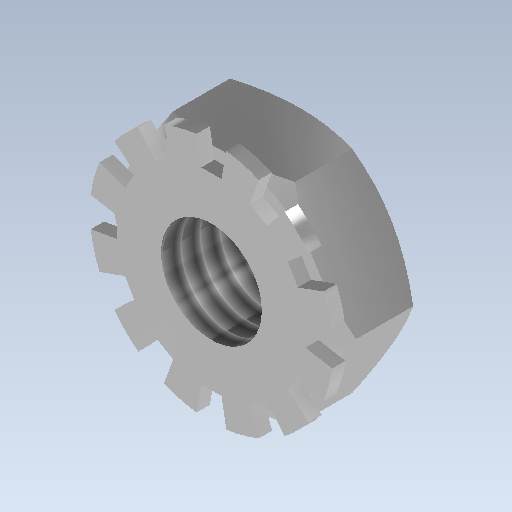
# Autodesk Inventor part: 275-1026
Saved by Autodesk Inventor 2020.2 (Build 242310000, 310)
## iProperties
Created: 2012-04-11
Part Number: 275-1026
Material: Stainless Steel, 440C
Document SubType Name: Modeling
Designer: Autodesk Inc.
Density: 7.75 g/cm^3
Catalog Web Link: http://www.vexrobotics.com/nuts-8-32.html
Vendor: VEX
Appearance: Black Chrome
Company: Autodesk Inc.
Category: Structure
Control State: 0
Master: False
Checked Out: False
Shininess: 70.0
Length Units: 11272
Angle Units: 11279
Time Units: 11290
Mass Units: 11286
Length Display Precision: 4
Angle Display Precision: 2
Compacted: True
Density: 7.75
Volumn: 0.07820028819372563
Area: 1.577785810948415
PropertySet Name: Model Information
Author: Autodesk Inc.
Autodesk Inventor part; units mm, degrees
ref_plane "YZ Plane" through (0, 0, 0) normal (1, 0, 0) x (0, 1, 0)
ref_plane "XZ Plane" through (0, 0, 0) normal (0, 1, 0) x (-1, 0, 0)
ref_plane "XY Plane" through (0, 0, 0) normal (0, 0, 1) x (1, 0, 0)
sketch "Sketch2" plane through (0, 0, 0) normal (0, 0, 1) x (1, 0, 0)
  circle A0 centre (0, 0) radius 5.0417 construction
  line L0 (-2.5209, 4.3663) -> (2.5209, 4.3663)
  line L1 (2.5209, 4.3663) -> (5.0417, 0)
  line L2 (5.0417, 0) -> (2.5209, -4.3663)
  line L3 (2.5209, -4.3663) -> (-2.5209, -4.3663)
  line L4 (-2.5209, -4.3663) -> (-5.0417, 0)
  line L5 (-5.0417, 0) -> (-2.5209, 4.3663)
  line L6 (0, 7.0584) -> (0, -7.0584) projected
  line L7 (-7.0584, 0) -> (7.0584, 0) projected
  dimension "Flats" = 8.7325
  constraints: 12 end point, 6 point on circle, 3 equal length, 2 midpoint, 1 centre point, 1 coincident, 1 parallel, 1 other
  measures "Flats" distance between parallel lines of L1 L4
extrude "Extrusion2" add sketch "Sketch2" along normal blind 3.1369
sketch "Sketch4" plane through (0, 0, 0) normal (1, 0, 0) x (0, 1, 0)
  line L0 (0, 3.1369) -> (4.3663, 3.1369) projected
  line L1 (4.3663, 3.1369) -> (8.7325, 0.616)
  line L2 (0, 0) -> (0, 3.1369) projected
  line L3 (4.3663, 3.1369) -> (8.7325, 3.1369)
  line L4 (8.7325, 0.616) -> (8.7325, 3.1369)
  dimension "d6" = 8.7325
  dimension "d7" = 30
  constraints: 6 end point, 2 perpendicular
  measures "d6" distance from line of L2 L1.end
  measures "d7" angle of L3 L1
revolve "Revolution1" cut sketch "Sketch4" angle 360 about axis through (0, 0, 0) along (0, 0, 1)
ref_plane "Work Plane1" through (0, 0, 1.5685) normal (0, 0, 1) x (1, 0, 0)
mirror "Mirror1" about plane through (0, 0, 1.5685) normal (0, 0, 1) of "Revolution1"
sketch "Sketch5" plane through (0, 0, 3.1369) normal (0, 0, 1) x (1, 0, 0)
  arc A0 (0, 4.3663) -> (-3.7813, 2.1831) centre (0, 0) ccw projected
  circle A1 centre (0, 0) radius 2.0828
  dimension "HoleDiam" = 4.1656
  constraints: 1 centre point, 1 coincident
  measures "HoleDiam" diameter of A1
extrude "Extrusion3" cut sketch "Sketch5" against normal through all
thread "Thread1" size "8-32 UNC" class "2B" standard "ANSI Unified Screw Threads" full length
sketch "Sketch7" plane through (0, 0, 3.1369) normal (0, 0, 1) x (1, 0, 0)
  circle A0 centre (0, 0) radius 2.0828 projected
  arc A1 (0, 4.3663) -> (-3.7813, 2.1831) centre (0, 0) ccw projected
  circle A2 centre (0, 0) radius 5.0212
  dimension "d18" = 10.0424
  constraints: 1 centre point, 1 coincident
  measures "d18" diameter of A2
extrude "Extrusion5" add sketch "Sketch7" along normal blind 0.5455
sketch "Sketch8" plane through (0, 0, 3.6824) normal (0, 0, 1) x (1, 0, 0)
  circle A0 centre (0, 0) radius 2.0828 projected
  line L0 (-0.611, 4.9839) -> (-0.4166, 3.8811)
  line L1 (-0.4166, 3.8811) -> (0.4166, 3.8811)
  line L2 (0.4166, 3.8811) -> (0.611, 4.9839)
  arc A1 (0.611, 4.9839) -> (-0.611, 4.9839) centre (0, 0) ccw
  circle A2 centre (0, 0) radius 5.0212 projected
  dimension "d21" = 100
  dimension "d22" = 100
  dimension "d23" = 3.8811
  dimension "d24" = 0.8331
  constraints: 6 end point, 2 concentric, 2 point on circle, 1 centre point, 1 equal length, 1 horizontal
  measures "d21" angle of L1 L0
  measures "d22" angle of L1 L2
  measures "d23" vertical distance of A0.centre L1.end
  measures "d24" distance of L0.end L1.end
extrude "Extrusion6" cut sketch "Sketch8" against normal blind 0.5455 contours A1 L2 L1 L0
pattern_circular "Circular Pattern1" count 12 over 360 about axis through (0, 0, 3.1369) along (0, 0, -1) of "Extrusion6"
equation "\"d6\" = Flats"
equation "\"d18\" = 1.15 * Flats"
equation "\"d19\" = 0.173913 * Height"
equation "\"d22\" = d21"
equation "\"d23\" = 0.444444 * Flats"
equation "\"d24\" = 0.2 * HoleDiam"
equation "\"d25\" = d19"
equation "\"Mirror_Plane\" = -0.5 * Height"
equation "\"Height\" = 3.1369"
body "Solid1"
